Autodesk Fusion 360 part; units mm, degrees
(part 3 of 4)
fillet "Fillet24" radius 0.2 24 edges at (33.2798, 72.3298, -1.0399) (37.5248, 72.3298, -1.45) (41.7697, 72.3298, -1.0399) (42.1798, 72.3298, 0.275) (41.7697, 72.3298, 1.5899) (37.5248, 72.3298, 2) (33.2798, 72.3298, 1.5899) (32.8698, 72.3298, 0.275) (24.1798, 72.3298, 0.275) (23.7697, 72.3298, -1.0399) (19.5248, 72.3298, -1.45) (15.2798, 72.3298, -1.0399) (14.8698, 72.3298, 0.275) (15.2798, 72.3298, 1.5899) (19.5248, 72.3298, 2) (23.7697, 72.3298, 1.5899) (50.5677, 72.3298, -1.9071) (57.5248, 72.3298, -2.2) (64.4819, 72.3298, -1.9071) (64.7748, 72.3298, 1.05) (64.4819, 72.3298, 4.0071) (57.5248, 72.3298, 4.3) (50.5677, 72.3298, 4.0071) (50.2748, 72.3298, 1.05) on bodies 1
sketch "Sketch11" plane through (0, 0, -5) normal (0, 0, -1) x (1, 0, 0)
  line L0 (-46.5752, 1.9808) -> (-75.3872, 18.6153)
  arc A0 (-75.9872, 19.6546) -> (-75.3872, 18.6153) centre (-74.7872, 19.6546) ccw
  line L1 (-75.9872, 19.6546) -> (-75.9872, 39.9015)
  arc A1 (-75.8268, 40.5008) -> (-75.9872, 39.9015) centre (-74.7872, 39.9015) ccw
  line L2 (-75.8268, 40.5008) -> (-59.4978, 68.8239)
  arc A2 (-57.8589, 69.2641) -> (-59.4978, 68.8239) centre (-58.4582, 68.2245) ccw
  line L3 (-57.8589, 69.2641) -> (-42.6922, 60.5201)
  line L4 (-41.6912, 54.388) -> (-12.2483, 37.4135)
  arc A3 (-11.6477, 36.3739) -> (-12.2483, 37.4135) centre (-12.8477, 36.3739) ccw
  line L5 (-11.6477, 36.3739) -> (-11.6477, 21.4833)
  line L6 (-11.2477, 20.7905) -> (-2.9111, 15.9774)
  line L7 (-2.5111, 15.8702) -> (29.0248, 15.8702)
  line L8 (29.8248, 16.6702) -> (29.8248, 18.6702)
  arc A4 (31.0248, 19.8702) -> (29.8248, 18.6702) centre (31.0248, 18.6702) ccw
  line L9 (31.0248, 19.8702) -> (67.0248, 19.8702)
  arc A5 (68.2248, 18.6702) -> (67.0248, 19.8702) centre (67.0248, 18.6702) ccw
  line L10 (68.2248, 18.6702) -> (68.2248, -69.3298)
  arc A6 (67.0248, -70.5298) -> (68.2248, -69.3298) centre (67.0248, -69.3298) ccw
  line L11 (67.0248, -70.5298) -> (-6.9752, -70.5298)
  arc A7 (-8.1752, -69.3298) -> (-6.9752, -70.5298) centre (-6.9752, -69.3298) ccw
  line L12 (-8.1752, -69.3298) -> (-8.1752, -58.3298)
  line L13 (-8.9752, -57.5298) -> (-27.1752, -57.5298)
  line L14 (-27.1752, -57.5298) -> (-27.1752, -55.3298)
  line L15 (-27.9752, -54.5298) -> (-44.9752, -54.5298)
  arc A8 (-46.1752, -53.3298) -> (-44.9752, -54.5298) centre (-44.9752, -53.3298) ccw
  line L16 (-46.1752, -53.3298) -> (-46.1752, 1.2879)
  line L17 (-35.3015, 58.3369) -> (-58.6925, 71.8224)
  line L18 (-60.0583, 71.4556) -> (-77.6535, 40.9362)
  line L19 (-77.7872, 40.4367) -> (-77.7872, 18.4999)
  line L20 (-77.2872, 17.6338) -> (-48.4752, 0.9993)
  line L21 (-47.9752, 0.1332) -> (-47.9752, -55.3298)
  line L22 (-46.9752, -56.3298) -> (-29.9752, -56.3298)
  line L23 (-28.9752, -57.3298) -> (-28.9752, -63.3298)
  line L24 (-9.9752, -65.3298) -> (-9.9752, -71.3298)
  line L25 (-8.9752, -72.3298) -> (69.0248, -72.3298)
  line L26 (70.0248, -71.3298) -> (70.0248, 20.6702)
  line L27 (69.0248, 21.6702) -> (25.0248, 21.6702)
  line L28 (23.0248, 17.6702) -> (-1.9752, 17.6702)
  line L29 (-2.4752, 17.8042) -> (-9.3477, 21.772)
  line L30 (-9.8477, 22.638) -> (-9.8477, 37.5294)
  line L31 (-10.3482, 38.3957) -> (-35.9725, 53.1687)
  line L32 (64.7748, -70.5298) -> (50.2748, -70.5298)
  line L33 (50.2748, -70.5298) -> (50.2748, -71.3298)
  line L34 (50.2748, -71.3298) -> (64.7748, -71.3298)
  line L35 (64.7748, -71.3298) -> (64.7748, -70.5298)
  line L36 (42.1798, -70.5298) -> (32.8698, -70.5298)
  line L37 (32.8698, -70.5298) -> (32.8698, -70.9298)
  line L38 (32.8698, -70.9298) -> (42.1798, -70.9298)
  line L39 (42.1798, -70.9298) -> (42.1798, -70.5298)
  line L40 (24.1798, -70.5298) -> (14.8698, -70.5298)
  line L41 (14.8698, -70.5298) -> (14.8698, -70.9298)
  line L42 (14.8698, -70.9298) -> (24.1798, -70.9298)
  line L43 (24.1798, -70.9298) -> (24.1798, -70.5298)
  line L44 (37.5248, -70.9298) -> (37.5248, -70.5298) construction
  line L45 (19.5248, -70.9298) -> (19.5248, -70.5298) construction
  line L46 (57.5248, -71.3298) -> (57.5248, -70.5298) construction
  arc A9 (-8.1752, -58.3298) -> (-8.9752, -57.5298) centre (-8.9752, -58.3298) ccw
  arc A10 (-27.1752, -55.3298) -> (-27.9752, -54.5298) centre (-27.9752, -55.3298) ccw
  arc A11 (-46.1752, 1.2879) -> (-46.5752, 1.9808) centre (-46.9752, 1.2879) ccw
  arc A12 (-11.6477, 21.4833) -> (-11.2477, 20.7905) centre (-10.8477, 21.4833) ccw
  arc A13 (-2.9111, 15.9774) -> (-2.5111, 15.8702) centre (-2.5111, 16.6702) ccw
  arc A14 (29.0248, 15.8702) -> (29.8248, 16.6702) centre (29.0248, 16.6702) ccw
  arc A15 (69.0248, -72.3298) -> (70.0248, -71.3298) centre (69.0248, -71.3298) ccw
  arc A16 (70.0248, 20.6702) -> (69.0248, 21.6702) centre (69.0248, 20.6702) ccw
  arc A17 (25.0248, 21.6702) -> (24.0248, 20.6702) centre (25.0248, 20.6702) ccw
  line L47 (24.0248, 20.6702) -> (24.0248, 18.6702)
  arc A18 (23.0248, 17.6702) -> (24.0248, 18.6702) centre (23.0248, 18.6702) ccw
  arc A19 (-2.4752, 17.8042) -> (-1.9752, 17.6702) centre (-1.9752, 18.6702) ccw
  arc A20 (-9.8477, 22.638) -> (-9.3477, 21.772) centre (-8.8477, 22.638) ccw
  arc A21 (-9.8477, 37.5294) -> (-10.3482, 38.3957) centre (-10.8477, 37.5294) ccw
  arc A22 (-36.3394, 54.5345) -> (-35.9725, 53.1687) centre (-35.473, 54.0351) ccw
  line L48 (-36.3394, 54.5345) -> (-34.9346, 56.9711)
  arc A23 (-34.9346, 56.9711) -> (-35.3015, 58.3369) centre (-35.8009, 57.4706) ccw
  arc A24 (-58.6925, 71.8224) -> (-60.0583, 71.4556) centre (-59.192, 70.9561) ccw
  arc A25 (-77.6535, 40.9362) -> (-77.7872, 40.4367) centre (-76.7872, 40.4367) ccw
  arc A26 (-77.7872, 18.4999) -> (-77.2872, 17.6338) centre (-76.7872, 18.4999) ccw
  arc A27 (-47.9752, 0.1332) -> (-48.4752, 0.9993) centre (-48.9752, 0.1332) ccw
  arc A28 (-47.9752, -55.3298) -> (-46.9752, -56.3298) centre (-46.9752, -55.3298) ccw
  arc A29 (-28.9752, -57.3298) -> (-29.9752, -56.3298) centre (-29.9752, -57.3298) ccw
  arc A30 (-28.9752, -63.3298) -> (-27.9752, -64.3298) centre (-27.9752, -63.3298) ccw
  line L49 (-27.9752, -64.3298) -> (-10.9752, -64.3298)
  arc A31 (-9.9752, -65.3298) -> (-10.9752, -64.3298) centre (-10.9752, -65.3298) ccw
  arc A32 (-9.9752, -71.3298) -> (-8.9752, -72.3298) centre (-8.9752, -71.3298) ccw
  line L50 (-42.0916, 59.4805) -> (-42.0916, 55.0811)
  arc A33 (-42.0916, 55.0811) -> (-41.6912, 54.388) centre (-41.2916, 55.0811) ccw
  arc A34 (-42.0916, 59.4805) -> (-42.6922, 60.5201) centre (-43.2916, 59.4805) ccw
  dimension "d187" = 18
  dimension "d188" = 20
  dimension "d189" = 14.5
  dimension "d190" = 9.31
  dimension "d192" = 12.5
  dimension "d193" = 0.4
  dimension "d194" = 0.8
  constraint horizontal L32
  constraint vertical L33
  constraint horizontal L34
  constraint vertical L35
  constraint coincident L11 L32.start
  constraint horizontal L36
  constraint vertical L37
  constraint horizontal L38
  constraint vertical L39
  constraint coincident L11 L36.start
  constraint horizontal L40
  constraint vertical L41
  constraint horizontal L42
  constraint vertical L43
  constraint coincident L11 L40.start
  constraint collinear L38 L42
  constraint midpoint L38 L44.start
  constraint midpoint L36 L44.end
  constraint perpendicular L11 L44
  constraint midpoint L42 L45.start
  constraint midpoint L40 L45.end
  constraint perpendicular L11 L45
  constraint midpoint L34 L46.start
  constraint midpoint L32 L46.end
  constraint equal L38 L42
  measures "d187" distance of L44 L45
  measures "d188" distance of L44 L46
  measures "d189" distance of L33.end L34.end
  measures "d190" distance of L37.end L38.end
  measures "d192" distance of L26 L46
  measures "d193" distance of L36 L38
  measures "d194" distance of L32 L34
extrude "Extrude12" cut sketch "Sketch11" against normal blind 5 contours L11 L40 L41 L42 L43 | L11 L36 L37 L38 L39 | L11 L32 L33 L34 L35 bodies 1
sketch "Sketch12" plane through (0, 0, -5) normal (0, 0, -1) x (1, 0, 0)
  line L0 (50.2748, -71.3298) -> (50.2748, -70.5298)
  line L1 (50.2748, -70.5298) -> (42.1798, -70.5298)
  line L2 (42.1798, -70.5298) -> (42.1798, -70.9298)
  line L3 (42.1798, -70.9298) -> (32.8698, -70.9298)
  line L4 (32.8698, -70.9298) -> (32.8698, -70.5298)
  line L5 (32.8698, -70.5298) -> (24.1798, -70.5298)
  line L6 (24.1798, -70.5298) -> (24.1798, -70.9298)
  line L7 (24.1798, -70.9298) -> (14.8698, -70.9298)
  line L8 (14.8698, -70.9298) -> (14.8698, -70.5298)
  line L9 (14.8698, -70.5298) -> (-6.9752, -70.5298)
  arc A0 (-8.1752, -69.3298) -> (-6.9752, -70.5298) centre (-6.9752, -69.3298) ccw
  line L10 (-8.1752, -69.3298) -> (-8.1752, -58.3298)
  arc A1 (-8.1752, -58.3298) -> (-8.9752, -57.5298) centre (-8.9752, -58.3298) ccw
  line L11 (-8.9752, -57.5298) -> (-27.1752, -57.5298)
  line L12 (-27.1752, -57.5298) -> (-27.1752, -55.3298)
  arc A2 (-27.1752, -55.3298) -> (-27.9752, -54.5298) centre (-27.9752, -55.3298) ccw
  line L13 (-27.9752, -54.5298) -> (-44.9752, -54.5298)
  arc A3 (-46.1752, -53.3298) -> (-44.9752, -54.5298) centre (-44.9752, -53.3298) ccw
  line L14 (-46.1752, -53.3298) -> (-46.1752, 1.2879)
  arc A4 (-46.1752, 1.2879) -> (-46.5752, 1.9808) centre (-46.9752, 1.2879) ccw
  line L15 (-46.5752, 1.9808) -> (-75.3872, 18.6153)
  arc A5 (-75.9872, 19.6546) -> (-75.3872, 18.6153) centre (-74.7872, 19.6546) ccw
  line L16 (-75.9872, 19.6546) -> (-75.9872, 39.9015)
  arc A6 (-75.8268, 40.5008) -> (-75.9872, 39.9015) centre (-74.7872, 39.9015) ccw
  line L17 (-75.8268, 40.5008) -> (-59.4978, 68.8239)
  arc A7 (-57.8589, 69.2641) -> (-59.4978, 68.8239) centre (-58.4582, 68.2245) ccw
  line L18 (-57.8589, 69.2641) -> (-42.6922, 60.5201)
  line L19 (-41.6912, 54.388) -> (-12.2483, 37.4135)
  arc A8 (-11.6477, 36.3739) -> (-12.2483, 37.4135) centre (-12.8477, 36.3739) ccw
  line L20 (-11.6477, 36.3739) -> (-11.6477, 21.4833)
  arc A9 (-11.6477, 21.4833) -> (-11.2477, 20.7905) centre (-10.8477, 21.4833) ccw
  line L21 (-11.2477, 20.7905) -> (-2.9111, 15.9774)
  arc A10 (-2.9111, 15.9774) -> (-2.5111, 15.8702) centre (-2.5111, 16.6702) ccw
  line L22 (-2.5111, 15.8702) -> (29.0248, 15.8702)
  arc A11 (29.0248, 15.8702) -> (29.8248, 16.6702) centre (29.0248, 16.6702) ccw
  line L23 (29.8248, 16.6702) -> (29.8248, 18.6702)
  arc A12 (31.0248, 19.8702) -> (29.8248, 18.6702) centre (31.0248, 18.6702) ccw
  line L24 (31.0248, 19.8702) -> (67.0248, 19.8702)
  arc A13 (68.2248, 18.6702) -> (67.0248, 19.8702) centre (67.0248, 18.6702) ccw
  line L25 (68.2248, 18.6702) -> (68.2248, -69.3298)
  arc A14 (67.0248, -70.5298) -> (68.2248, -69.3298) centre (67.0248, -69.3298) ccw
  line L26 (67.0248, -70.5298) -> (64.7748, -70.5298)
  line L27 (64.7748, -70.5298) -> (64.7748, -71.3298)
  line L28 (64.7748, -71.3298) -> (50.2748, -71.3298)
  arc A15 (69.0248, -72.3298) -> (70.0248, -71.3298) centre (69.0248, -71.3298) ccw
  line L29 (70.0248, -71.3298) -> (70.0248, 20.6702)
  arc A16 (70.0248, 20.6702) -> (69.0248, 21.6702) centre (69.0248, 20.6702) ccw
  line L30 (69.0248, 21.6702) -> (25.0248, 21.6702)
  arc A17 (25.0248, 21.6702) -> (24.0248, 20.6702) centre (25.0248, 20.6702) ccw
  line L31 (24.0248, 20.6702) -> (24.0248, 18.6702)
  arc A18 (23.0248, 17.6702) -> (24.0248, 18.6702) centre (23.0248, 18.6702) ccw
  line L32 (23.0248, 17.6702) -> (-1.9752, 17.6702)
  arc A19 (-2.4752, 17.8042) -> (-1.9752, 17.6702) centre (-1.9752, 18.6702) ccw
  line L33 (-2.4752, 17.8042) -> (-9.3477, 21.772)
  arc A20 (-9.8477, 22.638) -> (-9.3477, 21.772) centre (-8.8477, 22.638) ccw
  line L34 (-9.8477, 22.638) -> (-9.8477, 37.5294)
  arc A21 (-9.8477, 37.5294) -> (-10.3482, 38.3957) centre (-10.8477, 37.5294) ccw
  line L35 (-10.3482, 38.3957) -> (-35.9725, 53.1687)
  arc A22 (-36.3394, 54.5345) -> (-35.9725, 53.1687) centre (-35.473, 54.0351) ccw
  line L36 (-36.3394, 54.5345) -> (-34.9346, 56.9711)
  arc A23 (-34.9346, 56.9711) -> (-35.3015, 58.3369) centre (-35.8009, 57.4706) ccw
  line L37 (-35.3015, 58.3369) -> (-58.6925, 71.8224)
  arc A24 (-58.6925, 71.8224) -> (-60.0583, 71.4556) centre (-59.192, 70.9561) ccw
  line L38 (-60.0583, 71.4556) -> (-77.6535, 40.9362)
  arc A25 (-77.6535, 40.9362) -> (-77.7872, 40.4367) centre (-76.7872, 40.4367) ccw
  line L39 (-77.7872, 40.4367) -> (-77.7872, 18.4999)
  arc A26 (-77.7872, 18.4999) -> (-77.2872, 17.6338) centre (-76.7872, 18.4999) ccw
  line L40 (-77.2872, 17.6338) -> (-48.4752, 0.9993)
  arc A27 (-47.9752, 0.1332) -> (-48.4752, 0.9993) centre (-48.9752, 0.1332) ccw
  line L41 (-47.9752, 0.1332) -> (-47.9752, -55.3298)
  arc A28 (-47.9752, -55.3298) -> (-46.9752, -56.3298) centre (-46.9752, -55.3298) ccw
  line L42 (-46.9752, -56.3298) -> (-29.9752, -56.3298)
  arc A29 (-28.9752, -57.3298) -> (-29.9752, -56.3298) centre (-29.9752, -57.3298) ccw
  line L43 (-28.9752, -57.3298) -> (-28.9752, -63.3298)
  arc A30 (-28.9752, -63.3298) -> (-27.9752, -64.3298) centre (-27.9752, -63.3298) ccw
  line L44 (-27.9752, -64.3298) -> (-10.9752, -64.3298)
  arc A31 (-9.9752, -65.3298) -> (-10.9752, -64.3298) centre (-10.9752, -65.3298) ccw
  line L45 (-9.9752, -65.3298) -> (-9.9752, -71.3298)
  arc A32 (-9.9752, -71.3298) -> (-8.9752, -72.3298) centre (-8.9752, -71.3298) ccw
  line L46 (-8.9752, -72.3298) -> (69.0248, -72.3298)
  line L47 (-8.1752, -62.5298) -> (-27.1752, -62.5298)
  line L48 (-27.1752, -62.5298) -> (-27.1752, -57.5298)
  line L49 (-39.2973, 53.0078) -> (-36.8936, 57.1771)
  line L50 (-36.8936, 57.1771) -> (-42.6922, 60.5201)
  line L51 (31.0248, 19.8702) -> (25.8248, 19.8702)
  line L52 (25.8248, 19.8702) -> (25.8248, 15.8702)
  line L53 (-42.0916, 59.4805) -> (-42.0916, 55.0811)
  arc A33 (-42.0916, 59.4805) -> (-42.6922, 60.5201) centre (-43.2916, 59.4805) ccw
  arc A34 (-42.0916, 55.0811) -> (-41.6912, 54.388) centre (-41.2916, 55.0811) ccw
  dimension "d208" = 1.8
  dimension "d209" = 1.8
  dimension "d210" = 1.8
  constraint coincident L10 L47.start
  constraint perpendicular L10 L47
  constraint coincident L11.end L12.start
  constraint vertical L48
  constraint coincident L19 L49.start
  constraint perpendicular L19 L49
  constraint coincident L18.end L50.end
  constraint coincident A12.start L24.start
  constraint tangent A12 L51
  constraint perpendicular L51 L52
  constraint coincident L22 L52.end
  constraint perpendicular L49 L50
  measures "d208" distance of L31 L52
  measures "d209" distance of L36 L49
  measures "d210" distance of L44 L47
extrude "Extrude13" cut sketch "Sketch12" against normal blind 1.5 contours L22 A11 L23 A12 L51 L52 | L10 A1 L11 L47 L48 | L19 L49 L50 L53 A33 A34 bodies 1
fillet "Fillet27" radius 0.8 3 edges at (-39.2973, -53.0078, -4.25) (25.8248, -15.8702, -4.25) (-8.1752, 62.5298, -4.25) on bodies 1
sketch "Sketch13" plane through (0, 0, -3.5) normal (0, 0, -1) x (1, 0, 0)
  line L0 (-41.6912, 54.388) -> (-38.6042, 52.6083)
  arc A0 (-38.8977, 53.7009) -> (-38.6042, 52.6083) centre (-38.2046, 53.3013) ccw
  line L1 (-38.8977, 53.7009) -> (-36.8936, 57.1771)
  line L2 (-36.8936, 57.1771) -> (-42.6922, 60.5201)
  circle A1 centre (-40.2644, 56.3357) radius 1
  line L3 (-40.2644, 56.3357) -> (-43.2965, 58.0838) construction
  line L4 (-40.2644, 56.3357) -> (-41.4631, 54.2565) construction
  line L5 (-42.0916, 59.4805) -> (-42.0916, 55.0811)
  arc A2 (-42.0916, 55.0811) -> (-41.6912, 54.388) centre (-41.2916, 55.0811) ccw
  arc A3 (-42.0916, 59.4805) -> (-42.6922, 60.5201) centre (-43.2916, 59.4805) ccw
  dimension "d215" = 2
  dimension "d229" = 2.4
  dimension "d252" = 2.5
  constraint coincident A1.centre L3.start
  constraint coincident L0 L4.end
  constraint perpendicular L3 L4
  measures "d215" diameter of A1
  measures "d229" distance of L0 L3
  measures "d252" distance of L1 L4
extrude "Extrude14" cut sketch "Sketch13" against normal blind 4 contours A1 bodies 1
sketch "Sketch14" plane through (0, 0, -3.5) normal (0, 0, -1) x (1, 0, 0)
  line L0 (-8.1752, -63.3298) -> (-8.1752, -58.3298)
  arc A0 (-8.1752, -58.3298) -> (-8.9752, -57.5298) centre (-8.9752, -58.3298) ccw
  line L1 (-8.9752, -57.5298) -> (-27.1752, -57.5298)
  line L2 (-27.1752, -57.5298) -> (-27.1752, -62.5298)
  line L3 (-27.1752, -62.5298) -> (-8.9752, -62.5298)
  arc A1 (-8.1752, -63.3298) -> (-8.9752, -62.5298) centre (-8.9752, -63.3298) ccw
  circle A2 centre (-24.1752, -60.0298) radius 1
  line L4 (-24.1752, -60.0298) -> (-8.1752, -60.0298) construction
  line L5 (-24.1752, -60.0298) -> (-24.1752, -57.5298) construction
  dimension "d219" = 2
  dimension "d220" = 2.5
  dimension "d221" = 3
  constraint coincident A2.centre L4.start
  constraint coincident L0 L4.end
  constraint perpendicular L0 L4
  constraint coincident L1 L5.end
  constraint perpendicular L1 L5
  measures "d219" diameter of A2
  measures "d220" distance of A2.centre L5.end
  measures "d221" distance of L2 L5
extrude "Extrude15" cut sketch "Sketch14" against normal blind 4 contours A2 bodies 1
sketch "Sketch15" plane through (0, 0, -3.5) normal (0, 0, -1) x (1, 0, 0)
  line L0 (31.0248, 19.8702) -> (25.8248, 19.8702)
  line L1 (25.8248, 19.8702) -> (25.8248, 16.6702)
  arc A0 (25.0248, 15.8702) -> (25.8248, 16.6702) centre (25.0248, 16.6702) ccw
  line L2 (25.0248, 15.8702) -> (29.0248, 15.8702)
  arc A1 (29.0248, 15.8702) -> (29.8248, 16.6702) centre (29.0248, 16.6702) ccw
  line L3 (29.8248, 16.6702) -> (29.8248, 18.6702)
  arc A2 (31.0248, 19.8702) -> (29.8248, 18.6702) centre (31.0248, 18.6702) ccw
  circle A3 centre (27.8248, 17.8702) radius 1
  line L4 (27.8248, 17.8702) -> (27.8248, 15.8702) construction
  line L5 (27.8248, 17.8702) -> (29.8248, 17.8702) construction
  dimension "d224" = 2
  dimension "d225" = 2
  dimension "d226" = 2
  constraint coincident A3.centre L4.start
  constraint coincident L2 L4.end
  constraint perpendicular L2 L4
  constraint coincident L3 L5.end
  constraint perpendicular L3 L5
  measures "d224" diameter of A3
  measures "d225" distance of A3.centre L5.end
  measures "d226" distance of A3.centre L4.end
extrude "Extrude16" cut sketch "Sketch15" against normal blind 4 contours A3 bodies 1
sketch "Sketch16" plane through (0, 0, 0) normal (0, 0, -1) x (1, 0, 0)
  line L0 (32.8698, -70.5298) -> (32.8698, -63.3298)
  line L1 (32.8698, -63.3298) -> (42.1798, -63.3298)
  line L2 (42.1798, -63.3298) -> (42.1798, -70.5298)
  line L3 (42.1798, -70.5298) -> (50.2748, -70.5298)
  line L4 (50.2748, -70.5298) -> (50.2748, -57.3298)
  line L5 (50.2748, -57.3298) -> (64.7748, -57.3298)
  line L6 (64.7748, -57.3298) -> (64.7748, -70.5298)
  line L7 (64.7748, -70.5298) -> (67.0248, -70.5298)
  arc A0 (67.0248, -70.5298) -> (68.2248, -69.3298) centre (67.0248, -69.3298) ccw
  line L8 (68.2248, -69.3298) -> (68.2248, 18.6702)
  arc A1 (68.2248, 18.6702) -> (67.0248, 19.8702) centre (67.0248, 18.6702) ccw
  line L9 (67.0248, 19.8702) -> (31.0248, 19.8702)
  arc A2 (31.0248, 19.8702) -> (29.8248, 18.6702) centre (31.0248, 18.6702) ccw
  line L10 (29.8248, 18.6702) -> (29.8248, 16.6702)
  arc A3 (29.0248, 15.8702) -> (29.8248, 16.6702) centre (29.0248, 16.6702) ccw
  line L11 (29.0248, 15.8702) -> (-2.5111, 15.8702)
  arc A4 (-2.9111, 15.9774) -> (-2.5111, 15.8702) centre (-2.5111, 16.6702) ccw
  line L12 (-2.9111, 15.9774) -> (-11.2477, 20.7905)
  arc A5 (-11.6477, 21.4833) -> (-11.2477, 20.7905) centre (-10.8477, 21.4833) ccw
  line L13 (-11.6477, 21.4833) -> (-11.6477, 36.3739)
  arc A6 (-11.6477, 36.3739) -> (-12.2483, 37.4135) centre (-12.8477, 36.3739) ccw
  line L14 (-12.2483, 37.4135) -> (-41.6912, 54.388)
  line L15 (-42.6922, 60.5201) -> (-57.8589, 69.2641)
  arc A7 (-57.8589, 69.2641) -> (-59.4978, 68.8239) centre (-58.4582, 68.2245) ccw
  line L16 (-59.4978, 68.8239) -> (-75.8268, 40.5008)
  arc A8 (-75.8268, 40.5008) -> (-75.9872, 39.9015) centre (-74.7872, 39.9015) ccw
  line L17 (-75.9872, 39.9015) -> (-75.9872, 19.6546)
  arc A9 (-75.9872, 19.6546) -> (-75.3872, 18.6153) centre (-74.7872, 19.6546) ccw
  line L18 (-75.3872, 18.6153) -> (-46.5752, 1.9808)
  arc A10 (-46.1752, 1.2879) -> (-46.5752, 1.9808) centre (-46.9752, 1.2879) ccw
  line L19 (-46.1752, 1.2879) -> (-46.1752, -53.3298)
  arc A11 (-46.1752, -53.3298) -> (-44.9752, -54.5298) centre (-44.9752, -53.3298) ccw
  line L20 (-44.9752, -54.5298) -> (-27.9752, -54.5298)
  arc A12 (-27.1752, -55.3298) -> (-27.9752, -54.5298) centre (-27.9752, -55.3298) ccw
  line L21 (-27.1752, -55.3298) -> (-27.1752, -57.5298)
  line L22 (-27.1752, -57.5298) -> (-8.9752, -57.5298)
  arc A13 (-8.1752, -58.3298) -> (-8.9752, -57.5298) centre (-8.9752, -58.3298) ccw
  line L23 (-8.1752, -58.3298) -> (-8.1752, -69.3298)
  arc A14 (-8.1752, -69.3298) -> (-6.9752, -70.5298) centre (-6.9752, -69.3298) ccw
  line L24 (-6.9752, -70.5298) -> (14.8698, -70.5298)
  line L25 (14.8698, -70.5298) -> (14.8698, -63.3298)
  line L26 (14.8698, -63.3298) -> (24.1798, -63.3298)
  line L27 (24.1798, -63.3298) -> (24.1798, -70.5298)
  line L28 (24.1798, -70.5298) -> (32.8698, -70.5298)
  line L29 (-55.0372, 33.2941) -> (-55.0372, 19.2941)
  line L30 (-55.0372, 19.2941) -> (-71.0372, 19.2941)
  line L31 (-71.0372, 19.2941) -> (-71.0372, 33.2941)
  line L32 (-71.0372, 33.2941) -> (-55.0372, 33.2941)
  line L33 (-25.0752, -40.2298) -> (-9.8752, -40.2298)
  line L34 (-9.8752, -40.2298) -> (-9.8752, -55.4298)
  line L35 (-9.8752, -55.4298) -> (-25.0752, -55.4298)
  line L36 (-25.0752, -55.4298) -> (-25.0752, -40.2298)
  line L37 (-6.0752, -47.2298) -> (9.1248, -47.2298)
  line L38 (9.1248, -47.2298) -> (9.1248, -62.4298)
  line L39 (9.1248, -62.4298) -> (-6.0752, -62.4298)
  line L40 (-6.0752, -62.4298) -> (-6.0752, -47.2298)
  line L41 (31.9248, -20.2298) -> (47.1248, -20.2298)
  line L42 (47.1248, -20.2298) -> (47.1248, -35.4298)
  line L43 (47.1248, -35.4298) -> (31.9248, -35.4298)
  line L44 (31.9248, -35.4298) -> (31.9248, -20.2298)
  line L45 (50.9248, 2.5702) -> (50.9248, 17.7702)
  line L46 (50.9248, 17.7702) -> (66.1248, 17.7702)
  line L47 (66.1248, 17.7702) -> (66.1248, 2.5702)
  line L48 (66.1248, 2.5702) -> (50.9248, 2.5702)
  line L49 (12.9248, 13.7702) -> (28.1248, 13.7702)
  line L50 (28.1248, 13.7702) -> (28.1248, -1.4298)
  line L51 (28.1248, -1.4298) -> (12.9248, -1.4298)
  line L52 (12.9248, -1.4298) -> (12.9248, 13.7702)
  line L53 (-25.0752, 16.7702) -> (-9.8752, 16.7702)
  line L54 (-9.8752, 16.7702) -> (-9.8752, 1.5702)
  line L55 (-9.8752, 1.5702) -> (-25.0752, 1.5702)
  line L56 (-25.0752, 1.5702) -> (-25.0752, 16.7702)
  line L57 (-59.3299, 64.9107) -> (-46.1616, 57.3188)
  line L58 (-46.1616, 57.3188) -> (-53.7535, 44.1505)
  line L59 (-53.7535, 44.1505) -> (-66.9217, 51.7424)
  line L60 (-66.9217, 51.7424) -> (-59.3299, 64.9107)
  line L61 (-44.0752, 19.7702) -> (-28.8752, 19.7702)
  line L62 (-28.8752, 19.7702) -> (-28.8752, 4.5702)
  line L63 (-28.8752, 4.5702) -> (-44.0752, 4.5702)
  line L64 (-44.0752, 4.5702) -> (-44.0752, 19.7702)
  line L65 (-6.0752, 9.7702) -> (9.1248, 9.7702)
  line L66 (9.1248, 9.7702) -> (9.1248, -5.4298)
  line L67 (9.1248, -5.4298) -> (-6.0752, -5.4298)
  line L68 (-6.0752, -5.4298) -> (-6.0752, 9.7702)
  line L69 (31.9248, 2.5702) -> (31.9248, 17.7702)
  line L70 (31.9248, 17.7702) -> (47.1248, 17.7702)
  line L71 (47.1248, 17.7702) -> (47.1248, 2.5702)
  line L72 (47.1248, 2.5702) -> (31.9248, 2.5702)
  line L73 (50.9248, -20.2298) -> (66.1248, -20.2298)
  line L74 (66.1248, -20.2298) -> (66.1248, -35.4298)
  line L75 (66.1248, -35.4298) -> (50.9248, -35.4298)
  line L76 (50.9248, -35.4298) -> (50.9248, -20.2298)
  line L77 (-6.0752, -28.2298) -> (9.1248, -28.2298)
  line L78 (9.1248, -28.2298) -> (9.1248, -43.4298)
  line L79 (9.1248, -43.4298) -> (-6.0752, -43.4298)
  line L80 (-6.0752, -43.4298) -> (-6.0752, -28.2298)
  line L81 (-44.0752, -37.2298) -> (-28.8752, -37.2298)
  line L82 (-28.8752, -37.2298) -> (-28.8752, -52.4298)
  line L83 (-28.8752, -52.4298) -> (-44.0752, -52.4298)
  line L84 (-44.0752, -52.4298) -> (-44.0752, -37.2298)
  line L85 (-25.0752, -21.2298) -> (-9.8752, -21.2298)
  line L86 (-9.8752, -21.2298) -> (-9.8752, -36.4298)
  line L87 (-9.8752, -36.4298) -> (-25.0752, -36.4298)
  line L88 (-25.0752, -36.4298) -> (-25.0752, -21.2298)
  line L89 (12.9248, -24.2298) -> (28.1248, -24.2298)
  line L90 (28.1248, -24.2298) -> (28.1248, -39.4298)
  line L91 (28.1248, -39.4298) -> (12.9248, -39.4298)
  line L92 (12.9248, -39.4298) -> (12.9248, -24.2298)
  line L93 (31.9248, -39.2298) -> (47.1248, -39.2298)
  line L94 (47.1248, -39.2298) -> (47.1248, -54.4298)
  line L95 (47.1248, -54.4298) -> (31.9248, -54.4298)
  line L96 (31.9248, -54.4298) -> (31.9248, -39.2298)
  line L97 (50.9248, -1.2298) -> (66.1248, -1.2298)
  line L98 (66.1248, -1.2298) -> (66.1248, -16.4298)
  line L99 (66.1248, -16.4298) -> (50.9248, -16.4298)
  line L100 (50.9248, -16.4298) -> (50.9248, -1.2298)
  line L101 (-6.0752, -9.2298) -> (9.1248, -9.2298)
  line L102 (9.1248, -9.2298) -> (9.1248, -24.4298)
  line L103 (9.1248, -24.4298) -> (-6.0752, -24.4298)
  line L104 (-6.0752, -24.4298) -> (-6.0752, -9.2298)
  line L105 (-44.0752, -14.4298) -> (-44.0752, 0.7702)
  line L106 (-44.0752, 0.7702) -> (-28.8752, 0.7702)
  line L107 (-28.8752, 0.7702) -> (-28.8752, -14.4298)
  line L108 (-28.8752, -14.4298) -> (-44.0752, -14.4298)
  line L109 (-38.4949, 32.5761) -> (-51.6632, 40.1679)
  line L110 (-51.6632, 40.1679) -> (-44.0714, 53.3362)
  line L111 (-44.0714, 53.3362) -> (-30.9031, 45.7444)
  line L112 (-30.9031, 45.7444) -> (-38.4949, 32.5761)
  line L113 (-27.611, 43.8464) -> (-14.4427, 36.2546)
  line L114 (-14.4427, 36.2546) -> (-22.0346, 23.0863)
  line L115 (-22.0346, 23.0863) -> (-35.2029, 30.6781)
  line L116 (-35.2029, 30.6781) -> (-27.611, 43.8464)
  line L117 (-25.0752, -2.2298) -> (-9.8752, -2.2298)
  line L118 (-9.8752, -2.2298) -> (-9.8752, -17.4298)
  line L119 (-9.8752, -17.4298) -> (-25.0752, -17.4298)
  line L120 (-25.0752, -17.4298) -> (-25.0752, -2.2298)
  line L121 (12.9248, -5.2298) -> (28.1248, -5.2298)
  line L122 (28.1248, -5.2298) -> (28.1248, -20.4298)
  line L123 (28.1248, -20.4298) -> (12.9248, -20.4298)
  line L124 (12.9248, -20.4298) -> (12.9248, -5.2298)
  line L125 (31.9248, -1.2298) -> (47.1248, -1.2298)
  line L126 (47.1248, -1.2298) -> (47.1248, -16.4298)
  line L127 (47.1248, -16.4298) -> (31.9248, -16.4298)
  line L128 (31.9248, -16.4298) -> (31.9248, -1.2298)
  line L129 (50.9248, -39.2298) -> (66.1248, -39.2298)
  line L130 (66.1248, -39.2298) -> (66.1248, -54.4298)
  line L131 (66.1248, -54.4298) -> (50.9248, -54.4298)
  line L132 (50.9248, -54.4298) -> (50.9248, -39.2298)
  line L133 (12.9248, -43.2298) -> (28.1248, -43.2298)
  line L134 (28.1248, -43.2298) -> (28.1248, -58.4298)
  line L135 (28.1248, -58.4298) -> (12.9248, -58.4298)
  line L136 (12.9248, -58.4298) -> (12.9248, -43.2298)
  line L137 (-44.0752, -18.2298) -> (-28.8752, -18.2298)
  line L138 (-28.8752, -18.2298) -> (-28.8752, -33.4298)
  line L139 (-28.8752, -33.4298) -> (-44.0752, -33.4298)
  line L140 (-44.0752, -33.4298) -> (-44.0752, -18.2298)
  line L141 (44.1798, -70.5298) -> (30.8698, -70.5298)
  line L142 (30.8698, -70.5298) -> (30.8698, -62.3294)
  line L143 (30.8698, -62.3294) -> (44.1798, -62.3294)
  line L144 (44.1798, -62.3294) -> (44.1798, -70.5298)
  line L145 (26.1798, -70.5298) -> (12.8698, -70.5298)
  line L146 (12.8698, -70.5298) -> (12.8698, -62.3294)
  line L147 (12.8698, -62.3294) -> (26.1798, -62.3294)
  line L148 (26.1798, -62.3294) -> (26.1798, -70.5298)
  line L149 (66.7748, -70.5298) -> (48.2748, -70.5298)
  line L150 (48.2748, -70.5298) -> (48.2748, -56.3298)
  line L151 (48.2748, -56.3298) -> (66.7748, -56.3298)
  line L152 (66.7748, -56.3298) -> (66.7748, -70.5298)
  line L153 (-42.0916, 55.0811) -> (-42.0916, 59.4805)
  arc A15 (-42.0916, 55.0811) -> (-41.6912, 54.388) centre (-41.2916, 55.0811) ccw
  arc A16 (-42.0916, 59.4805) -> (-42.6922, 60.5201) centre (-43.2916, 59.4805) ccw
  dimension "d230" = 2
  dimension "d231" = 2
  dimension "d232" = 2
  dimension "d233" = 2
  dimension "d234" = 1.0004
  dimension "d235" = 2
  dimension "d236" = 2
  dimension "d237" = 1
  constraint horizontal L141
  constraint vertical L142
  constraint horizontal L143
  constraint vertical L144
  constraint coincident L3 L141.start
  constraint horizontal L145
  constraint vertical L146
  constraint horizontal L147
  constraint vertical L148
  constraint coincident L28 L145.start
  constraint horizontal L149
  constraint vertical L150
  constraint horizontal L151
  constraint vertical L152
  constraint coincident L7 L149.start
  constraint collinear L143 L147
  measures "d230" distance of L2 L144
  measures "d231" distance of L0 L142
  measures "d232" distance of L27 L148
  measures "d233" distance of L25 L146
  measures "d234" distance of L1 L143
  measures "d235" distance of L4 L150
  measures "d236" distance of L6 L152
  measures "d237" distance of L5 L151
extrude "Extrude17" cut sketch "Sketch16" against normal blind 1 contours L0 L1 L2 L3 L28 L141 L142 L143 L144 | L24 L25 L26 L27 L28 L145 L146 L147 L148 | L3 L4 L5 L6 L7 L149 L150 L151 L152 bodies 1
fillet "Fillet28" radius 1 36 edges at (69.7319, -21.3773, -5) (47.0248, -21.6702, -5) (24.3177, -21.3773, -5) (24.0248, -19.6702, -5) (23.7319, -17.9631, -5) (10.5248, -17.6702, -5) (-2.2341, -17.7043, -5) (-5.9115, -19.7881, -5) (-9.7137, -22.138, -5) (-9.8477, -30.0837, -5) (-9.9818, -38.0297, -5) (-23.1604, -45.7822, -5) (-36.4388, -53.7757, -5) (-35.637, -55.7528, -5) (-34.8352, -57.73, -5) (-46.997, -65.0797, -5) (-59.4514, -71.9219, -5) (-68.8559, -56.1959, -5) (-77.7532, -40.6952, -5) (-77.7872, -29.4683, -5) (-77.6532, -17.9999, -5) (-62.8812, -9.3166, -5) (-48.1092, -0.6332, -5) (-47.9752, 27.5983, -5) (-47.6823, 56.0369, -5) (-38.4752, 56.3298, -5) (-29.2681, 56.6227, -5) (-28.9752, 60.3298, -5) (-28.6823, 64.0369, -5) (-19.4752, 64.3298, -5) (-10.2681, 64.6227, -5) (-9.9752, 68.3298, -5) (-9.6823, 72.0369, -5) (30.0248, 72.3298, -5) (69.7319, 72.0369, -5) (70.0248, 25.3298, -5) on bodies 1
sketch "Sketch17" plane through (0, 0, 2.5) normal (0, 0, 1) x (-1, 0, 0)
  line L0 (-48.7748, -57.3298) -> (-48.7748, -71.3298)
  line L1 (-48.7748, -71.3298) -> (-43.3798, -71.3298)
  line L2 (-43.3798, -71.3298) -> (-43.3798, -61.1298)
  line L3 (-43.3798, -61.1298) -> (-31.6698, -61.1298)
  line L4 (-31.6698, -61.1298) -> (-31.6698, -71.3298)
  line L5 (-31.6698, -71.3298) -> (-25.3798, -71.3298)
  line L6 (-25.3798, -71.3298) -> (-25.3798, -61.1298)
  line L7 (-25.3798, -61.1298) -> (-13.6698, -61.1298)
  line L8 (-13.6698, -61.1298) -> (-13.6698, -71.3298)
  line L9 (-13.6698, -71.3298) -> (8.9752, -71.3298)
  line L10 (8.9752, -71.3298) -> (8.9752, -65.3298)
  arc A0 (10.9752, -63.3298) -> (8.9752, -65.3298) centre (10.9752, -65.3298) ccw
  line L11 (10.9752, -63.3298) -> (27.9752, -63.3298)
  line L12 (27.9752, -63.3298) -> (27.9752, -57.3298)
  arc A1 (29.9752, -55.3298) -> (27.9752, -57.3298) centre (29.9752, -57.3298) ccw
  line L13 (29.9752, -55.3298) -> (46.9752, -55.3298)
  line L14 (46.9752, -55.3298) -> (46.9752, 0.1332)
  arc A2 (47.9752, 1.8653) -> (46.9752, 0.1332) centre (48.9752, 0.1332) ccw
  line L15 (47.9752, 1.8653) -> (76.7872, 18.4999)
  line L16 (76.7872, 18.4999) -> (76.7872, 40.4367)
  line L17 (76.7872, 40.4367) -> (59.192, 70.9561)
  line L18 (59.192, 70.9561) -> (35.8009, 57.4706)
  line L19 (35.8009, 57.4706) -> (37.2057, 55.034)
  arc A3 (36.4719, 52.3024) -> (37.2057, 55.034) centre (35.473, 54.0351) ccw
  line L20 (36.4719, 52.3024) -> (10.8477, 37.5294)
  line L21 (10.8477, 37.5294) -> (10.8477, 22.638)
  arc A4 (9.8477, 20.906) -> (10.8477, 22.638) centre (8.8477, 22.638) ccw
  line L22 (9.8477, 20.906) -> (2.9752, 16.9381)
  arc A5 (1.9752, 16.6702) -> (2.9752, 16.9381) centre (1.9752, 18.6702) ccw
  line L23 (1.9752, 16.6702) -> (-23.0248, 16.6702)
  arc A6 (-25.0248, 18.6702) -> (-23.0248, 16.6702) centre (-23.0248, 18.6702) ccw
  line L24 (-25.0248, 18.6702) -> (-25.0248, 20.6702)
  line L25 (-25.0248, 20.6702) -> (-69.0248, 20.6702)
  line L26 (-69.0248, 20.6702) -> (-69.0248, -71.3298)
  line L27 (-69.0248, -71.3298) -> (-66.2748, -71.3298)
  line L28 (-66.2748, -71.3298) -> (-66.2748, -57.3298)
  arc A7 (-65.2748, -56.3298) -> (-66.2748, -57.3298) centre (-65.2748, -57.3298) ccw
  line L29 (-65.2748, -56.3298) -> (-49.7748, -56.3298)
  arc A8 (-48.7748, -57.3298) -> (-49.7748, -56.3298) centre (-49.7748, -57.3298) ccw
  line L30 (-14.4248, -38.9298) -> (-26.6248, -38.9298)
  arc A9 (-27.6248, -37.9298) -> (-26.6248, -38.9298) centre (-26.6248, -37.9298) ccw
  line L31 (-27.6248, -37.9298) -> (-27.6248, -25.7298)
  arc A10 (-26.6248, -24.7298) -> (-27.6248, -25.7298) centre (-26.6248, -25.7298) ccw
  line L32 (-26.6248, -24.7298) -> (-14.4248, -24.7298)
  arc A11 (-13.4248, -25.7298) -> (-14.4248, -24.7298) centre (-14.4248, -25.7298) ccw
  line L33 (-13.4248, -25.7298) -> (-13.4248, -37.9298)
  arc A12 (-14.4248, -38.9298) -> (-13.4248, -37.9298) centre (-14.4248, -37.9298) ccw
  line L34 (-52.4248, 3.0702) -> (-64.6248, 3.0702)
  arc A13 (-65.6248, 4.0702) -> (-64.6248, 3.0702) centre (-64.6248, 4.0702) ccw
  line L35 (-65.6248, 4.0702) -> (-65.6248, 16.2702)
  arc A14 (-64.6248, 17.2702) -> (-65.6248, 16.2702) centre (-64.6248, 16.2702) ccw
  line L36 (-64.6248, 17.2702) -> (-52.4248, 17.2702)
  arc A15 (-51.4248, 16.2702) -> (-52.4248, 17.2702) centre (-52.4248, 16.2702) ccw
  line L37 (-51.4248, 16.2702) -> (-51.4248, 4.0702)
  arc A16 (-52.4248, 3.0702) -> (-51.4248, 4.0702) centre (-52.4248, 4.0702) ccw
  line L38 (50.114, 39.8519) -> (39.5447, 33.7585)
  arc A17 (38.1789, 34.1253) -> (39.5447, 33.7585) centre (39.0452, 34.6248) ccw
  line L39 (38.1789, 34.1253) -> (32.0854, 44.6946)
  arc A18 (32.4523, 46.0604) -> (32.0854, 44.6946) centre (32.9518, 45.1941) ccw
  line L40 (32.4523, 46.0604) -> (43.0216, 52.1539)
  arc A19 (44.3874, 51.787) -> (43.0216, 52.1539) centre (43.5211, 51.2875) ccw
  line L41 (44.3874, 51.787) -> (50.4809, 41.2177)
  arc A20 (50.114, 39.8519) -> (50.4809, 41.2177) centre (49.6145, 40.7182) ccw
  line L42 (33.6536, 30.3621) -> (23.0843, 24.2686)
  arc A21 (21.7185, 24.6355) -> (23.0843, 24.2686) centre (22.5849, 25.135) ccw
  line L43 (21.7185, 24.6355) -> (15.6251, 35.2048)
  arc A22 (15.992, 36.5706) -> (15.6251, 35.2048) centre (16.4914, 35.7043) ccw
  line L44 (15.992, 36.5706) -> (26.5612, 42.6641)
  arc A23 (27.927, 42.2972) -> (26.5612, 42.6641) centre (27.0607, 41.7977) ccw
  line L45 (27.927, 42.2972) -> (34.0205, 31.7279)
  arc A24 (33.6536, 30.3621) -> (34.0205, 31.7279) centre (33.1542, 31.2284) ccw
  line L46 (-52.4248, -34.9298) -> (-64.6248, -34.9298)
  arc A25 (-65.6248, -33.9298) -> (-64.6248, -34.9298) centre (-64.6248, -33.9298) ccw
  line L47 (-65.6248, -33.9298) -> (-65.6248, -21.7298)
  arc A26 (-64.6248, -20.7298) -> (-65.6248, -21.7298) centre (-64.6248, -21.7298) ccw
  line L48 (-64.6248, -20.7298) -> (-52.4248, -20.7298)
  arc A27 (-51.4248, -21.7298) -> (-52.4248, -20.7298) centre (-52.4248, -21.7298) ccw
  line L49 (-51.4248, -21.7298) -> (-51.4248, -33.9298)
  arc A28 (-52.4248, -34.9298) -> (-51.4248, -33.9298) centre (-52.4248, -33.9298) ccw
  line L50 (-33.4248, -34.9298) -> (-45.6248, -34.9298)
  arc A29 (-46.6248, -33.9298) -> (-45.6248, -34.9298) centre (-45.6248, -33.9298) ccw
  line L51 (-46.6248, -33.9298) -> (-46.6248, -21.7298)
  arc A30 (-45.6248, -20.7298) -> (-46.6248, -21.7298) centre (-45.6248, -21.7298) ccw
  line L52 (-45.6248, -20.7298) -> (-33.4248, -20.7298)
  arc A31 (-32.4248, -21.7298) -> (-33.4248, -20.7298) centre (-33.4248, -21.7298) ccw
  line L53 (-32.4248, -21.7298) -> (-32.4248, -33.9298)
  arc A32 (-33.4248, -34.9298) -> (-32.4248, -33.9298) centre (-33.4248, -33.9298) ccw
  line L54 (42.5752, -32.9298) -> (30.3752, -32.9298)
  arc A33 (29.3752, -31.9298) -> (30.3752, -32.9298) centre (30.3752, -31.9298) ccw
  line L55 (29.3752, -31.9298) -> (29.3752, -19.7298)
  arc A34 (30.3752, -18.7298) -> (29.3752, -19.7298) centre (30.3752, -19.7298) ccw
  line L56 (30.3752, -18.7298) -> (42.5752, -18.7298)
  arc A35 (43.5752, -19.7298) -> (42.5752, -18.7298) centre (42.5752, -19.7298) ccw
  line L57 (43.5752, -19.7298) -> (43.5752, -31.9298)
  arc A36 (42.5752, -32.9298) -> (43.5752, -31.9298) centre (42.5752, -31.9298) ccw
  line L58 (4.5752, -23.9298) -> (-7.6248, -23.9298)
  arc A37 (-8.6248, -22.9298) -> (-7.6248, -23.9298) centre (-7.6248, -22.9298) ccw
  line L59 (-8.6248, -22.9298) -> (-8.6248, -10.7298)
  arc A38 (-7.6248, -9.7298) -> (-8.6248, -10.7298) centre (-7.6248, -10.7298) ccw
  line L60 (-7.6248, -9.7298) -> (4.5752, -9.7298)
  arc A39 (5.5752, -10.7298) -> (4.5752, -9.7298) centre (4.5752, -10.7298) ccw
  line L61 (5.5752, -10.7298) -> (5.5752, -22.9298)
  arc A40 (4.5752, -23.9298) -> (5.5752, -22.9298) centre (4.5752, -22.9298) ccw
  line L62 (-33.4248, 3.0702) -> (-45.6248, 3.0702)
  arc A41 (-46.6248, 4.0702) -> (-45.6248, 3.0702) centre (-45.6248, 4.0702) ccw
  line L63 (-46.6248, 4.0702) -> (-46.6248, 16.2702)
  arc A42 (-45.6248, 17.2702) -> (-46.6248, 16.2702) centre (-45.6248, 16.2702) ccw
  line L64 (-45.6248, 17.2702) -> (-33.4248, 17.2702)
  arc A43 (-32.4248, 16.2702) -> (-33.4248, 17.2702) centre (-33.4248, 16.2702) ccw
  line L65 (-32.4248, 16.2702) -> (-32.4248, 4.0702)
  arc A44 (-33.4248, 3.0702) -> (-32.4248, 4.0702) centre (-33.4248, 4.0702) ccw
  line L66 (65.3725, 51.4263) -> (54.8032, 45.3329)
  arc A45 (53.4374, 45.6998) -> (54.8032, 45.3329) centre (54.3038, 46.1992) ccw
  line L67 (53.4374, 45.6998) -> (47.344, 56.269)
  arc A46 (47.7108, 57.6348) -> (47.344, 56.269) centre (48.2103, 56.7685) ccw
  line L68 (47.7108, 57.6348) -> (58.2801, 63.7283)
  arc A47 (59.6459, 63.3614) -> (58.2801, 63.7283) centre (58.7796, 62.862) ccw
  line L69 (59.6459, 63.3614) -> (65.7394, 52.7921)
  arc A48 (65.3725, 51.4263) -> (65.7394, 52.7921) centre (64.873, 52.2927) ccw
  line L70 (-52.4248, -53.9298) -> (-64.6248, -53.9298)
  arc A49 (-65.6248, -52.9298) -> (-64.6248, -53.9298) centre (-64.6248, -52.9298) ccw
  line L71 (-65.6248, -52.9298) -> (-65.6248, -40.7298)
  arc A50 (-64.6248, -39.7298) -> (-65.6248, -40.7298) centre (-64.6248, -40.7298) ccw
  line L72 (-64.6248, -39.7298) -> (-52.4248, -39.7298)
  arc A51 (-51.4248, -40.7298) -> (-52.4248, -39.7298) centre (-52.4248, -40.7298) ccw
  line L73 (-51.4248, -40.7298) -> (-51.4248, -52.9298)
  arc A52 (-52.4248, -53.9298) -> (-51.4248, -52.9298) centre (-52.4248, -52.9298) ccw
  line L74 (23.5752, 2.0702) -> (11.3752, 2.0702)
  arc A53 (10.3752, 3.0702) -> (11.3752, 2.0702) centre (11.3752, 3.0702) ccw
  line L75 (10.3752, 3.0702) -> (10.3752, 15.2702)
  arc A54 (11.3752, 16.2702) -> (10.3752, 15.2702) centre (11.3752, 15.2702) ccw
  line L76 (11.3752, 16.2702) -> (23.5752, 16.2702)
  arc A55 (24.5752, 15.2702) -> (23.5752, 16.2702) centre (23.5752, 15.2702) ccw
  line L77 (24.5752, 15.2702) -> (24.5752, 3.0702)
  arc A56 (23.5752, 2.0702) -> (24.5752, 3.0702) centre (23.5752, 3.0702) ccw
  line L78 (42.5752, -13.9298) -> (30.3752, -13.9298)
  arc A57 (29.3752, -12.9298) -> (30.3752, -13.9298) centre (30.3752, -12.9298) ccw
  line L79 (29.3752, -12.9298) -> (29.3752, -0.7298)
  arc A58 (30.3752, 0.2702) -> (29.3752, -0.7298) centre (30.3752, -0.7298) ccw
  line L80 (30.3752, 0.2702) -> (42.5752, 0.2702)
  arc A59 (43.5752, -0.7298) -> (42.5752, 0.2702) centre (42.5752, -0.7298) ccw
  line L81 (43.5752, -0.7298) -> (43.5752, -12.9298)
  arc A60 (42.5752, -13.9298) -> (43.5752, -12.9298) centre (42.5752, -12.9298) ccw
  line L82 (42.5752, -51.9298) -> (30.3752, -51.9298)
  arc A61 (29.3752, -50.9298) -> (30.3752, -51.9298) centre (30.3752, -50.9298) ccw
  line L83 (29.3752, -50.9298) -> (29.3752, -38.7298)
  arc A62 (30.3752, -37.7298) -> (29.3752, -38.7298) centre (30.3752, -38.7298) ccw
  line L84 (30.3752, -37.7298) -> (42.5752, -37.7298)
  arc A63 (43.5752, -38.7298) -> (42.5752, -37.7298) centre (42.5752, -38.7298) ccw
  line L85 (43.5752, -38.7298) -> (43.5752, -50.9298)
  arc A64 (42.5752, -51.9298) -> (43.5752, -50.9298) centre (42.5752, -50.9298) ccw
  line L86 (4.5752, -4.9298) -> (-7.6248, -4.9298)
  arc A65 (-8.6248, -3.9298) -> (-7.6248, -4.9298) centre (-7.6248, -3.9298) ccw
  line L87 (-8.6248, -3.9298) -> (-8.6248, 8.2702)
  arc A66 (-7.6248, 9.2702) -> (-8.6248, 8.2702) centre (-7.6248, 8.2702) ccw
  line L88 (-7.6248, 9.2702) -> (4.5752, 9.2702)
  arc A67 (5.5752, 8.2702) -> (4.5752, 9.2702) centre (4.5752, 8.2702) ccw
  line L89 (5.5752, 8.2702) -> (5.5752, -3.9298)
  arc A68 (4.5752, -4.9298) -> (5.5752, -3.9298) centre (4.5752, -3.9298) ccw
  line L90 (23.5752, -16.9298) -> (11.3752, -16.9298)
  arc A69 (10.3752, -15.9298) -> (11.3752, -16.9298) centre (11.3752, -15.9298) ccw
  line L91 (10.3752, -15.9298) -> (10.3752, -3.7298)
  arc A70 (11.3752, -2.7298) -> (10.3752, -3.7298) centre (11.3752, -3.7298) ccw
  line L92 (11.3752, -2.7298) -> (23.5752, -2.7298)
  arc A71 (24.5752, -3.7298) -> (23.5752, -2.7298) centre (23.5752, -3.7298) ccw
  line L93 (24.5752, -3.7298) -> (24.5752, -15.9298)
  arc A72 (23.5752, -16.9298) -> (24.5752, -15.9298) centre (23.5752, -15.9298) ccw
  line L94 (-14.4248, -19.9298) -> (-26.6248, -19.9298)
  arc A73 (-27.6248, -18.9298) -> (-26.6248, -19.9298) centre (-26.6248, -18.9298) ccw
  line L95 (-27.6248, -18.9298) -> (-27.6248, -6.7298)
  arc A74 (-26.6248, -5.7298) -> (-27.6248, -6.7298) centre (-26.6248, -6.7298) ccw
  line L96 (-26.6248, -5.7298) -> (-14.4248, -5.7298)
  arc A75 (-13.4248, -6.7298) -> (-14.4248, -5.7298) centre (-14.4248, -6.7298) ccw
  line L97 (-13.4248, -6.7298) -> (-13.4248, -18.9298)
  arc A76 (-14.4248, -19.9298) -> (-13.4248, -18.9298) centre (-14.4248, -18.9298) ccw
  line L98 (-14.4248, -0.9298) -> (-26.6248, -0.9298)
  arc A77 (-27.6248, 0.0702) -> (-26.6248, -0.9298) centre (-26.6248, 0.0702) ccw
  line L99 (-27.6248, 0.0702) -> (-27.6248, 12.2702)
  arc A78 (-26.6248, 13.2702) -> (-27.6248, 12.2702) centre (-26.6248, 12.2702) ccw
  line L100 (-26.6248, 13.2702) -> (-14.4248, 13.2702)
  arc A79 (-13.4248, 12.2702) -> (-14.4248, 13.2702) centre (-14.4248, 12.2702) ccw
  line L101 (-13.4248, 12.2702) -> (-13.4248, 0.0702)
  arc A80 (-14.4248, -0.9298) -> (-13.4248, 0.0702) centre (-14.4248, 0.0702) ccw
  line L102 (23.5752, -35.9298) -> (11.3752, -35.9298)
  arc A81 (10.3752, -34.9298) -> (11.3752, -35.9298) centre (11.3752, -34.9298) ccw
  line L103 (10.3752, -34.9298) -> (10.3752, -22.7298)
  arc A82 (11.3752, -21.7298) -> (10.3752, -22.7298) centre (11.3752, -22.7298) ccw
  line L104 (11.3752, -21.7298) -> (23.5752, -21.7298)
  arc A83 (24.5752, -22.7298) -> (23.5752, -21.7298) centre (23.5752, -22.7298) ccw
  line L105 (24.5752, -22.7298) -> (24.5752, -34.9298)
  arc A84 (23.5752, -35.9298) -> (24.5752, -34.9298) centre (23.5752, -34.9298) ccw
  line L106 (4.5752, -61.9298) -> (-7.6248, -61.9298)
  arc A85 (-8.6248, -60.9298) -> (-7.6248, -61.9298) centre (-7.6248, -60.9298) ccw
  line L107 (-8.6248, -60.9298) -> (-8.6248, -48.7298)
  arc A86 (-7.6248, -47.7298) -> (-8.6248, -48.7298) centre (-7.6248, -48.7298) ccw
  line L108 (-7.6248, -47.7298) -> (4.5752, -47.7298)
  arc A87 (5.5752, -48.7298) -> (4.5752, -47.7298) centre (4.5752, -48.7298) ccw
  line L109 (5.5752, -48.7298) -> (5.5752, -60.9298)
  arc A88 (4.5752, -61.9298) -> (5.5752, -60.9298) centre (4.5752, -60.9298) ccw
  line L110 (-52.4248, -15.9298) -> (-64.6248, -15.9298)
  arc A89 (-65.6248, -14.9298) -> (-64.6248, -15.9298) centre (-64.6248, -14.9298) ccw
  line L111 (-65.6248, -14.9298) -> (-65.6248, -2.7298)
  arc A90 (-64.6248, -1.7298) -> (-65.6248, -2.7298) centre (-64.6248, -2.7298) ccw
  line L112 (-64.6248, -1.7298) -> (-52.4248, -1.7298)
  arc A91 (-51.4248, -2.7298) -> (-52.4248, -1.7298) centre (-52.4248, -2.7298) ccw
  line L113 (-51.4248, -2.7298) -> (-51.4248, -14.9298)
  arc A92 (-52.4248, -15.9298) -> (-51.4248, -14.9298) centre (-52.4248, -14.9298) ccw
  line L114 (-14.4248, -57.9298) -> (-26.6248, -57.9298)
  arc A93 (-27.6248, -56.9298) -> (-26.6248, -57.9298) centre (-26.6248, -56.9298) ccw
  line L115 (-27.6248, -56.9298) -> (-27.6248, -44.7298)
  arc A94 (-26.6248, -43.7298) -> (-27.6248, -44.7298) centre (-26.6248, -44.7298) ccw
  line L116 (-26.6248, -43.7298) -> (-14.4248, -43.7298)
  arc A95 (-13.4248, -44.7298) -> (-14.4248, -43.7298) centre (-14.4248, -44.7298) ccw
  line L117 (-13.4248, -44.7298) -> (-13.4248, -56.9298)
  arc A96 (-14.4248, -57.9298) -> (-13.4248, -56.9298) centre (-14.4248, -56.9298) ccw
  line L118 (-33.4248, -15.9298) -> (-45.6248, -15.9298)
  arc A97 (-46.6248, -14.9298) -> (-45.6248, -15.9298) centre (-45.6248, -14.9298) ccw
  line L119 (-46.6248, -14.9298) -> (-46.6248, -2.7298)
  arc A98 (-45.6248, -1.7298) -> (-46.6248, -2.7298) centre (-45.6248, -2.7298) ccw
  line L120 (-45.6248, -1.7298) -> (-33.4248, -1.7298)
  arc A99 (-32.4248, -2.7298) -> (-33.4248, -1.7298) centre (-33.4248, -2.7298) ccw
  line L121 (-32.4248, -2.7298) -> (-32.4248, -14.9298)
  arc A100 (-33.4248, -15.9298) -> (-32.4248, -14.9298) centre (-33.4248, -14.9298) ccw
  line L122 (4.5752, -42.9298) -> (-7.6248, -42.9298)
  arc A101 (-8.6248, -41.9298) -> (-7.6248, -42.9298) centre (-7.6248, -41.9298) ccw
  line L123 (-8.6248, -41.9298) -> (-8.6248, -29.7298)
  arc A102 (-7.6248, -28.7298) -> (-8.6248, -29.7298) centre (-7.6248, -29.7298) ccw
  line L124 (-7.6248, -28.7298) -> (4.5752, -28.7298)
  arc A103 (5.5752, -29.7298) -> (4.5752, -28.7298) centre (4.5752, -29.7298) ccw
  line L125 (5.5752, -29.7298) -> (5.5752, -41.9298)
  arc A104 (4.5752, -42.9298) -> (5.5752, -41.9298) centre (4.5752, -41.9298) ccw
  line L126 (-33.4248, -53.9298) -> (-45.6248, -53.9298)
  arc A105 (-46.6248, -52.9298) -> (-45.6248, -53.9298) centre (-45.6248, -52.9298) ccw
  line L127 (-46.6248, -52.9298) -> (-46.6248, -40.7298)
  arc A106 (-45.6248, -39.7298) -> (-46.6248, -40.7298) centre (-45.6248, -40.7298) ccw
  line L128 (-45.6248, -39.7298) -> (-33.4248, -39.7298)
  arc A107 (-32.4248, -40.7298) -> (-33.4248, -39.7298) centre (-33.4248, -40.7298) ccw
  line L129 (-32.4248, -40.7298) -> (-32.4248, -52.9298)
  arc A108 (-33.4248, -53.9298) -> (-32.4248, -52.9298) centre (-33.4248, -52.9298) ccw
  line L130 (42.5752, 5.0702) -> (30.3752, 5.0702)
  arc A109 (29.3752, 6.0702) -> (30.3752, 5.0702) centre (30.3752, 6.0702) ccw
  line L131 (29.3752, 6.0702) -> (29.3752, 18.2702)
  arc A110 (30.3752, 19.2702) -> (29.3752, 18.2702) centre (30.3752, 18.2702) ccw
  line L132 (30.3752, 19.2702) -> (42.5752, 19.2702)
  arc A111 (43.5752, 18.2702) -> (42.5752, 19.2702) centre (42.5752, 18.2702) ccw
  line L133 (43.5752, 18.2702) -> (43.5752, 6.0702)
  arc A112 (42.5752, 5.0702) -> (43.5752, 6.0702) centre (42.5752, 6.0702) ccw
  line L134 (68.4872, 20.2441) -> (58.0872, 20.2441)
  arc A113 (57.0872, 21.2441) -> (58.0872, 20.2441) centre (58.0872, 21.2441) ccw
  line L135 (57.0872, 21.2441) -> (57.0872, 31.3441)
  arc A114 (58.0872, 32.3441) -> (57.0872, 31.3441) centre (58.0872, 31.3441) ccw
  line L136 (58.0872, 32.3441) -> (68.4872, 32.3441)
  arc A115 (69.4872, 31.3441) -> (68.4872, 32.3441) centre (68.4872, 31.3441) ccw
  line L137 (69.4872, 31.3441) -> (69.4872, 21.2441)
  arc A116 (68.4872, 20.2441) -> (69.4872, 21.2441) centre (68.4872, 21.2441) ccw
  line L138 (23.5752, -54.9298) -> (11.3752, -54.9298)
  arc A117 (10.3752, -53.9298) -> (11.3752, -54.9298) centre (11.3752, -53.9298) ccw
  line L139 (10.3752, -53.9298) -> (10.3752, -41.7298)
  arc A118 (11.3752, -40.7298) -> (10.3752, -41.7298) centre (11.3752, -41.7298) ccw
  line L140 (11.3752, -40.7298) -> (23.5752, -40.7298)
  arc A119 (24.5752, -41.7298) -> (23.5752, -40.7298) centre (23.5752, -41.7298) ccw
  line L141 (24.5752, -41.7298) -> (24.5752, -53.9298)
  arc A120 (23.5752, -54.9298) -> (24.5752, -53.9298) centre (23.5752, -53.9298) ccw
  line L142 (59.059, 12.306) -> (62.309, 6.6768)
  line L143 (62.309, 6.6768) -> (61.443, 6.1768)
  line L144 (61.443, 6.1768) -> (58.193, 11.806)
  line L145 (58.193, 11.806) -> (59.059, 12.306)
  line L146 (56.0736, 3.0768) -> (52.8236, 8.706)
  line L147 (52.8236, 8.706) -> (51.9576, 8.206)
  line L148 (51.9576, 8.206) -> (55.2076, 2.5768)
  line L149 (55.2076, 2.5768) -> (56.0736, 3.0768)
  dimension "d242" = 3.5
  dimension "d243" = 1
  dimension "d246" = 19.45
  dimension "d247" = 3
  dimension "d248" = 1
  dimension "d249" = 3
  dimension "d250" = 3.5
  dimension "d251" = 7.2
  constraint perpendicular L15 L142
  constraint perpendicular L142 L143
  constraint perpendicular L15 L144
  constraint parallel L15 L145
  constraint perpendicular L15 L146
  constraint perpendicular L146 L147
  constraint perpendicular L15 L148
  constraint parallel L147 L149
  measures "d242" distance of L15 L145
  measures "d243" distance of L142.end L143.end
  measures "d246" distance of L15.end L144
  measures "d247" distance of L15 L143
  measures "d248" distance of L148.end L146.start
  measures "d249" distance of L15 L149
  measures "d250" distance of L15 L147
  measures "d251" distance of L144 L148
extrude "Extrude18" cut sketch "Sketch17" against normal blind 2.5 contours L15 L146 L147 L148 | L15 L146 L148 L149 | L15 L142 L144 L145 | L15 L142 L143 L144 bodies 1
fillet "Fillet29" radius 1.2 3 edges at (-36.8936, -57.1771, -4.25) (25.8248, -19.8702, -4.25) (-27.1752, 62.5298, -4.25) on bodies 1
mirror "Mirror1" about plane through (-77.7872, -40.7043, 0) normal (-1, 0, 0) of bodies 1 makes body 2
move_body "Move1" bodies 2 to x (1, 0, 0) y (0, 1, 0) z (0, 0, 1) at (-20, 0, 0)
equation "d1 = ( 4 * 19 ) * 1 mm"
equation "d2 = ( 2 * 19 ) * 1 mm"
equation "d3 = d1"
equation "d7 = d3"
equation "d10 = d7"
equation "d11 = d10"
equation "d43 = d42"
equation "d82 = d103"
equation "d83 = d103"
equation "d84 = d103"
equation "d85 = d103"
equation "d86 = d103"
equation "d87 = d103"
equation "d88 = d103"
equation "d89 = d103"
equation "d90 = d103"
equation "d91 = d103"
equation "d92 = d103"
equation "d93 = d103"
equation "d94 = d103"
equation "d95 = d103"
equation "d96 = d103"
equation "d97 = d103"
equation "d98 = d103"
equation "d99 = d103"
equation "d100 = d103"
equation "d101 = d103"